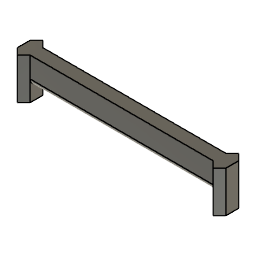
card-dispenser (Autodesk Fusion 360 archive; units mm, degrees)
design "dispenser-gate"
part number: 2026-07-27-01-31-44-288
Autodesk Fusion 360 part; units mm, degrees
(part 1 of 3)
sketch "Sketch1" plane through (0, 0, 0) normal (0, 0, 1) x (1, 0, 0)
  line L0 (0, 5) -> (5, 5)
  line L1 (5, 5) -> (5, 0)
  line L2 (5, 0) -> (0, 0)
  line L3 (0, 0) -> (0, 5)
  line L4 (0, 5) -> (2.5, 7.5)
  line L5 (2.5, 7.5) -> (5, 5)
  line L6 (0, 0) -> (2.5, -2.5)
  line L7 (2.5, -2.5) -> (5, 0)
  line L8 (0, 0) -> (81, 0)
  line L9 (81, 0) -> (81, 5)
  line L10 (81, 5) -> (0, 5)
  line L11 (81, 5) -> (76, 5)
  line L12 (76, 5) -> (76, 0)
  line L13 (76, 5) -> (78.5, 7.5)
  line L14 (78.5, 7.5) -> (81, 5)
  line L15 (81, 0) -> (78.5, -2.5)
  line L16 (76, 0) -> (78.5, -2.5)
  constraint horizontal L0
  constraint vertical L1
  constraint horizontal L2
  constraint vertical L3
  constraint perpendicular L4 L5
  constraint coincident L2.end L3.start
  constraint parallel L5 L6
  constraint perpendicular L6 L7
  constraint perpendicular L3 L8
  constraint perpendicular L2 L9
  constraint perpendicular L3 L10
  constraint coincident L10 L11.end
  constraint coincident L8 L12.end
  constraint perpendicular L8 L12
  constraint perpendicular L13 L14
  constraint perpendicular L14 L15
  constraint perpendicular L15 L16
extrude "Extrude1" add sketch "Sketch1" along normal blind 16
sketch "Sketch2" plane through (0, 0, 0) normal (0, -1, 0) x (1, 0, 0)
  line L0 (5, 0) -> (76, 0)
  line L1 (76, 0) -> (76, 16)
  line L2 (76, 16) -> (5, 16)
  line L3 (5, 16) -> (5, 0)
  line L4 (5, 0) -> (76, 0)
  line L5 (76, 0) -> (76, 5.45)
  line L6 (76, 5.45) -> (5, 5.45)
  line L7 (5, 5.45) -> (5, 0)
  dimension "d3" = 71
  dimension "d4" = 5.45
  constraint horizontal L4
  constraint vertical L5
  constraint horizontal L6
  constraint vertical L7
  constraint coincident L0.start L3.end
  measures "d3" distance of L0.start L0.end
  measures "d4" distance of L0.start L6.end
extrude "Extrude2" cut sketch "Sketch2" against normal blind 5 contours L0 L1 L3 L4 L5 L6 L7
fillet "Fillet1" radius 2.5 2 edges at (40.5, 0, 5.45) (40.5, 5, 5.45)

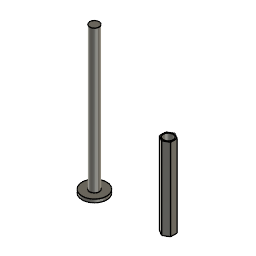
design "card-dispenser-shaft"
part number: 2026-07-26-23-05-58-167
part number: 2026-07-27-03-40-20-627
part number: 2026-07-27-03-40-25-472
Autodesk Fusion 360 part; units mm, degrees
sketch "Sketch1" plane through (0, 0, 0) normal (0, 0, 1) x (1, 0, 0)
  circle A0 centre (0, 0) radius 2.9
  circle A1 centre (0, 0) radius 7.5
  circle A2 centre (45, 0) radius 2.95
  line L0 (45, 4) -> (41.5359, 2)
  line L1 (41.5359, 2) -> (41.5359, -2)
  line L2 (41.5359, -2) -> (45, -4)
  line L3 (45, -4) -> (48.4641, -2)
  line L4 (48.4641, -2) -> (48.4641, 2)
  line L5 (48.4641, 2) -> (45, 4)
  point P0 (45, 0)
  point P1 (45, 0)
  dimension "d1" = 5.8
  dimension "d4" = 15
  dimension "d7" = 5.9
  constraint coincident A0.centre A1.centre
  constraint concentric A0 A1
  constraint coincident P1 P0
  measures "d1" diameter of A0
  measures "d4" diameter of A1
  measures "d7" diameter of A2
extrude "Extrude1" add sketch "Sketch1" along normal blind 87 contours A0 makes body 1
extrude "Extrude2" add sketch "Sketch1" against normal blind 2 contours A0 | A1 bodies 1
extrude "Extrude3" add sketch "Sketch1" along normal blind 50 separate body contours L0 L1 L2 L3 L4 L5 makes body 2
copy_body "Body->Comp1" bodies 2 removing the originals makes body 3 in component "Component"
copy_body "Body->Comp2" bodies 1 removing the originals makes body 4 in component "Component'"
component "Component" placed x (1, 0, 0) y (0, 1, 0) z (0, 0, 1) at (0, 0, 0)
component "Component'" placed x (1, 0, 0) y (0, 1, 0) z (0, 0, 1) at (0, 0, 0)

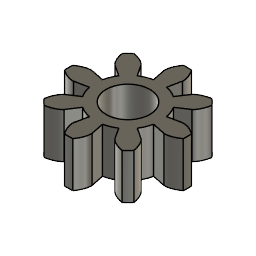
design "dispenser-driven-gear"
part number: 2026-07-25-20-51-35-213
part number: 2026-07-27-03-07-20-434
Autodesk Fusion 360 part; units mm, degrees
sketch "Sketch1" plane through (0, 0, 0) normal (0, 0, 1) x (1, 0, 0) in component "Component"
  spline S0 degree 5 poles (6.0079, -1.2297) (6.008, -1.2297) (6.0082, -1.2298) (6.0085, -1.2298) (6.009, -1.2299) (6.0098, -1.23) (6.0106, -1.2302) (6.0116, -1.2304) (6.0127, -1.2305) (6.0139, -1.2307) (6.0152, -1.2309) (6.0166, -1.2311) (6.0182, -1.2314) (6.0198, -1.2316) (6.0216, -1.2318) (6.0234, -1.2321) (6.0254, -1.2323) (6.0274, -1.2326) (6.0296, -1.2328) (6.0318, -1.2331) (6.0342, -1.2333) (6.0366, -1.2336) (6.0392, -1.2339) (6.0418, -1.2341) (6.0446, -1.2344) (6.0474, -1.2346) (6.0503, -1.2349) (6.0533, -1.2351) (6.0564, -1.2353) (6.0596, -1.2356) (6.0629, -1.2358) (6.0663, -1.236) (6.0698, -1.2362) (6.0733, -1.2364) (6.077, -1.2366) (6.0807, -1.2368) (6.0845, -1.237) (6.0884, -1.2371) (6.0923, -1.2373) (6.0964, -1.2374) (6.1005, -1.2375) (6.1047, -1.2376) (6.109, -1.2377) (6.1134, -1.2378) (6.1179, -1.2379) (6.1224, -1.2379) (6.127, -1.2379) (6.1317, -1.2379) (6.1364, -1.2379) (6.1413, -1.2379) (6.1462, -1.2379) (6.1511, -1.2378) (6.1562, -1.2377) (6.1613, -1.2376) (6.1665, -1.2375) (6.1718, -1.2373) (6.1771, -1.2372) (6.1825, -1.237) (6.188, -1.2367) (6.1935, -1.2365) (6.1991, -1.2362) (6.2048, -1.236) (6.2105, -1.2356) (6.2163, -1.2353) (6.2222, -1.2349) (6.2281, -1.2346) (6.2341, -1.2341) (6.2402, -1.2337) (6.2463, -1.2332) (6.2525, -1.2327) (6.2587, -1.2322) (6.265, -1.2317) (6.2714, -1.2311) (6.2778, -1.2305) (6.2843, -1.2299) (6.2909, -1.2292) (6.2975, -1.2285) (6.3041, -1.2278) (6.3109, -1.227) (6.3176, -1.2262) (6.3245, -1.2254) (6.3314, -1.2246) (6.3383, -1.2237) (6.3453, -1.2228) (6.3524, -1.2219) (6.3595, -1.2209) (6.3666, -1.2199) (6.3739, -1.2188) (6.3811, -1.2178) (6.3885, -1.2167) (6.3958, -1.2155) (6.4033, -1.2144) (6.4107, -1.2131) (6.4183, -1.2119) (6.4258, -1.2106) (6.4335, -1.2093) (6.4411, -1.208) (6.4489, -1.2066) (6.4566, -1.2052) (6.4645, -1.2037) (6.4723, -1.2022) (6.4802, -1.2007) (6.4882, -1.1991) (6.4962, -1.1975) (6.5043, -1.1959) (6.5124, -1.1942) (6.5205, -1.1925) (6.5287, -1.1908) (6.5369, -1.189) (6.5452, -1.1872) (6.5535, -1.1853) (6.5619, -1.1834) (6.5703, -1.1814) (6.5787, -1.1795) (6.5872, -1.1774) (6.5957, -1.1754) (6.6043, -1.1733) (6.6129, -1.1712) (6.6216, -1.169) (6.6302, -1.1668) (6.639, -1.1645) (6.6477, -1.1622) (6.6565, -1.1599) (6.6654, -1.1575) (6.6743, -1.1551) (6.6832, -1.1526) (6.6921, -1.1501) (6.7011, -1.1476) (6.7102, -1.145) (6.7192, -1.1424) (6.7283, -1.1397) (6.7375, -1.137) (6.7466, -1.1342) (6.7558, -1.1314) (6.7651, -1.1286) (6.7744, -1.1257) (6.7837, -1.1228) (6.793, -1.1199) (6.8024, -1.1168) (6.8118, -1.1138) (6.8212, -1.1107) (6.8307, -1.1076) (6.8402, -1.1044) (6.8497, -1.1012) (6.8593, -1.0979) (6.8689, -1.0946) (6.8785, -1.0913) (6.8881, -1.0879) (6.8978, -1.0844) (6.9075, -1.0809) (6.9173, -1.0774) (6.927, -1.0738) (6.9368, -1.0702) (6.9467, -1.0666) (6.9565, -1.0628) (6.9664, -1.0591) (6.9763, -1.0553) (6.9862, -1.0515) (6.9962, -1.0476) (7.0062, -1.0436) (7.0162, -1.0397) (7.0262, -1.0356) (7.0363, -1.0316) (7.0464, -1.0275) (7.0565, -1.0233) (7.0666, -1.0191) (7.0768, -1.0149) (7.087, -1.0106) (7.0972, -1.0062) (7.1074, -1.0018) (7.1176, -0.9974) (7.1279, -0.9929) (7.1382, -0.9884) (7.1485, -0.9838) (7.1589, -0.9792) (7.1692, -0.9745) (7.1796, -0.9698) (7.19, -0.9651) (7.2004, -0.9603) (7.2109, -0.9554) (7.2213, -0.9505) (7.2318, -0.9456) (7.2423, -0.9406) (7.2528, -0.9356) (7.2634, -0.9305) (7.2739, -0.9253) (7.2845, -0.9202) (7.2951, -0.9149) (7.3057, -0.9097) (7.3163, -0.9044) (7.327, -0.899) (7.3376, -0.8936) (7.3483, -0.8881) (7.359, -0.8826) (7.3697, -0.8771) (7.3804, -0.8714) (7.3912, -0.8658) (7.4019, -0.8601) (7.4127, -0.8544) (7.4235, -0.8486) (7.4343, -0.8427) (7.4451, -0.8368) (7.4559, -0.8309) (7.4667, -0.8249) (7.4776, -0.8189) (7.4885, -0.8128) (7.4993, -0.8067) (7.5102, -0.8005) (7.5211, -0.7943) (7.532, -0.788) (7.543, -0.7817) (7.5539, -0.7753) (7.5648, -0.7689) (7.5758, -0.7624) (7.5868, -0.7559) (7.5978, -0.7494) (7.6087, -0.7428) (7.6197, -0.7361) (7.6308, -0.7294) (7.6418, -0.7226) (7.6528, -0.7158) (7.6638, -0.709) (7.6749, -0.7021) (7.6859, -0.6951) (7.697, -0.6882) (7.7081, -0.6811) (7.7192, -0.674) (7.7302, -0.6669) (7.7413, -0.6597) (7.7524, -0.6525) (7.7635, -0.6452) (7.7746, -0.6378) (7.7858, -0.6305) (7.7969, -0.623) (7.808, -0.6156) (7.8192, -0.608) (7.8303, -0.6005) (7.8415, -0.5928) (7.8526, -0.5852) (7.8638, -0.5774) (7.8749, -0.5697) (7.8839, -0.5634) (7.8906, -0.5587) (7.895, -0.5556) (7.8973, -0.554) knots 0 0 0 0 0 0 0.00416667 0.00833333 0.0125 0.01666667 0.02083333 0.025 0.02916667 0.03333333 0.0375 0.04166667 0.04583333 0.05 0.05416667 0.05833333 0.0625 0.06666667 0.07083333 0.075 0.07916667 0.08333333 0.0875 0.09166667 0.09583333 0.1 0.10416667 0.10833333 0.1125 0.11666667 0.12083333 0.125 0.12916667 0.13333333 0.1375 0.14166667 0.14583333 0.15 0.15416667 0.15833333 0.1625 0.16666667 0.17083333 0.175 0.17916667 0.18333333 0.1875 0.19166667 0.19583333 0.2 0.20416667 0.20833333 0.2125 0.21666667 0.22083333 0.225 0.22916667 0.23333333 0.2375 0.24166667 0.24583333 0.25 0.25416667 0.25833333 0.2625 0.26666667 0.27083333 0.275 0.27916667 0.28333333 0.2875 0.29166667 0.29583333 0.3 0.30416667 0.30833333 0.3125 0.31666667 0.32083333 0.325 0.32916667 0.33333333 0.3375 0.34166667 0.34583333 0.35 0.35416667 0.35833333 0.3625 0.36666667 0.37083333 0.375 0.37916667 0.38333333 0.3875 0.39166667 0.39583333 0.4 0.40416667 0.40833333 0.4125 0.41666667 0.42083333 0.425 0.42916667 0.43333333 0.4375 0.44166667 0.44583333 0.45 0.45416667 0.45833333 0.4625 0.46666667 0.47083333 0.475 0.47916667 0.48333333 0.4875 0.49166667 0.49583333 0.5 0.50416667 0.50833333 0.5125 0.51666667 0.52083333 0.525 0.52916667 0.53333333 0.5375 0.54166667 0.54583333 0.55 0.55416667 0.55833333 0.5625 0.56666667 0.57083333 0.575 0.57916667 0.58333333 0.5875 0.59166667 0.59583333 0.6 0.60416667 0.60833333 0.6125 0.61666667 0.62083333 0.625 0.62916667 0.63333333 0.6375 0.64166667 0.64583333 0.65 0.65416667 0.65833333 0.6625 0.66666667 0.67083333 0.675 0.67916667 0.68333333 0.6875 0.69166667 0.69583333 0.7 0.70416667 0.70833333 0.7125 0.71666667 0.72083333 0.725 0.72916667 0.73333333 0.7375 0.74166667 0.74583333 0.75 0.75416667 0.75833333 0.7625 0.76666667 0.77083333 0.775 0.77916667 0.78333333 0.7875 0.79166667 0.79583333 0.8 0.80416667 0.80833333 0.8125 0.81666667 0.82083333 0.825 0.82916667 0.83333333 0.8375 0.84166667 0.84583333 0.85 0.85416667 0.85833333 0.8625 0.86666667 0.87083333 0.875 0.87916667 0.88333333 0.8875 0.89166667 0.89583333 0.9 0.90416667 0.90833333 0.9125 0.91666667 0.92083333 0.925 0.92916667 0.93333333 0.9375 0.94166667 0.94583333 0.95 0.95416667 0.95833333 0.9625 0.96666667 0.97083333 0.975 0.97916667 0.98333333 0.9875 0.99166667 0.99583333 1 1 1 1 1 1
  spline S1 degree 5 poles (6.0079, 1.2297) (6.008, 1.2297) (6.0082, 1.2298) (6.0085, 1.2298) (6.009, 1.2299) (6.0098, 1.23) (6.0106, 1.2302) (6.0116, 1.2304) (6.0127, 1.2305) (6.0139, 1.2307) (6.0152, 1.2309) (6.0166, 1.2311) (6.0182, 1.2314) (6.0198, 1.2316) (6.0216, 1.2318) (6.0234, 1.2321) (6.0254, 1.2323) (6.0274, 1.2326) (6.0296, 1.2328) (6.0318, 1.2331) (6.0342, 1.2333) (6.0366, 1.2336) (6.0392, 1.2339) (6.0418, 1.2341) (6.0446, 1.2344) (6.0474, 1.2346) (6.0503, 1.2349) (6.0533, 1.2351) (6.0564, 1.2353) (6.0596, 1.2356) (6.0629, 1.2358) (6.0663, 1.236) (6.0698, 1.2362) (6.0733, 1.2364) (6.077, 1.2366) (6.0807, 1.2368) (6.0845, 1.237) (6.0884, 1.2371) (6.0923, 1.2373) (6.0964, 1.2374) (6.1005, 1.2375) (6.1047, 1.2376) (6.109, 1.2377) (6.1134, 1.2378) (6.1179, 1.2379) (6.1224, 1.2379) (6.127, 1.2379) (6.1317, 1.2379) (6.1364, 1.2379) (6.1413, 1.2379) (6.1462, 1.2379) (6.1511, 1.2378) (6.1562, 1.2377) (6.1613, 1.2376) (6.1665, 1.2375) (6.1718, 1.2373) (6.1771, 1.2372) (6.1825, 1.237) (6.188, 1.2367) (6.1935, 1.2365) (6.1991, 1.2362) (6.2048, 1.236) (6.2105, 1.2356) (6.2163, 1.2353) (6.2222, 1.2349) (6.2281, 1.2346) (6.2341, 1.2341) (6.2402, 1.2337) (6.2463, 1.2332) (6.2525, 1.2327) (6.2587, 1.2322) (6.265, 1.2317) (6.2714, 1.2311) (6.2778, 1.2305) (6.2843, 1.2299) (6.2909, 1.2292) (6.2975, 1.2285) (6.3041, 1.2278) (6.3109, 1.227) (6.3176, 1.2262) (6.3245, 1.2254) (6.3314, 1.2246) (6.3383, 1.2237) (6.3453, 1.2228) (6.3524, 1.2219) (6.3595, 1.2209) (6.3666, 1.2199) (6.3739, 1.2188) (6.3811, 1.2178) (6.3885, 1.2167) (6.3958, 1.2155) (6.4033, 1.2144) (6.4107, 1.2131) (6.4183, 1.2119) (6.4258, 1.2106) (6.4335, 1.2093) (6.4411, 1.208) (6.4489, 1.2066) (6.4566, 1.2052) (6.4645, 1.2037) (6.4723, 1.2022) (6.4802, 1.2007) (6.4882, 1.1991) (6.4962, 1.1975) (6.5043, 1.1959) (6.5124, 1.1942) (6.5205, 1.1925) (6.5287, 1.1908) (6.5369, 1.189) (6.5452, 1.1872) (6.5535, 1.1853) (6.5619, 1.1834) (6.5703, 1.1814) (6.5787, 1.1795) (6.5872, 1.1774) (6.5957, 1.1754) (6.6043, 1.1733) (6.6129, 1.1712) (6.6216, 1.169) (6.6302, 1.1668) (6.639, 1.1645) (6.6477, 1.1622) (6.6565, 1.1599) (6.6654, 1.1575) (6.6743, 1.1551) (6.6832, 1.1526) (6.6921, 1.1501) (6.7011, 1.1476) (6.7102, 1.145) (6.7192, 1.1424) (6.7283, 1.1397) (6.7375, 1.137) (6.7466, 1.1342) (6.7558, 1.1314) (6.7651, 1.1286) (6.7744, 1.1257) (6.7837, 1.1228) (6.793, 1.1199) (6.8024, 1.1168) (6.8118, 1.1138) (6.8212, 1.1107) (6.8307, 1.1076) (6.8402, 1.1044) (6.8497, 1.1012) (6.8593, 1.0979) (6.8689, 1.0946) (6.8785, 1.0913) (6.8881, 1.0879) (6.8978, 1.0844) (6.9075, 1.0809) (6.9173, 1.0774) (6.927, 1.0738) (6.9368, 1.0702) (6.9467, 1.0666) (6.9565, 1.0628) (6.9664, 1.0591) (6.9763, 1.0553) (6.9862, 1.0515) (6.9962, 1.0476) (7.0062, 1.0436) (7.0162, 1.0397) (7.0262, 1.0356) (7.0363, 1.0316) (7.0464, 1.0275) (7.0565, 1.0233) (7.0666, 1.0191) (7.0768, 1.0149) (7.087, 1.0106) (7.0972, 1.0062) (7.1074, 1.0018) (7.1176, 0.9974) (7.1279, 0.9929) (7.1382, 0.9884) (7.1485, 0.9838) (7.1589, 0.9792) (7.1692, 0.9745) (7.1796, 0.9698) (7.19, 0.9651) (7.2004, 0.9603) (7.2109, 0.9554) (7.2213, 0.9505) (7.2318, 0.9456) (7.2423, 0.9406) (7.2528, 0.9356) (7.2634, 0.9305) (7.2739, 0.9253) (7.2845, 0.9202) (7.2951, 0.9149) (7.3057, 0.9097) (7.3163, 0.9044) (7.327, 0.899) (7.3376, 0.8936) (7.3483, 0.8881) (7.359, 0.8826) (7.3697, 0.8771) (7.3804, 0.8714) (7.3912, 0.8658) (7.4019, 0.8601) (7.4127, 0.8544) (7.4235, 0.8486) (7.4343, 0.8427) (7.4451, 0.8368) (7.4559, 0.8309) (7.4667, 0.8249) (7.4776, 0.8189) (7.4885, 0.8128) (7.4993, 0.8067) (7.5102, 0.8005) (7.5211, 0.7943) (7.532, 0.788) (7.543, 0.7817) (7.5539, 0.7753) (7.5648, 0.7689) (7.5758, 0.7624) (7.5868, 0.7559) (7.5978, 0.7494) (7.6087, 0.7428) (7.6197, 0.7361) (7.6308, 0.7294) (7.6418, 0.7226) (7.6528, 0.7158) (7.6638, 0.709) (7.6749, 0.7021) (7.6859, 0.6951) (7.697, 0.6882) (7.7081, 0.6811) (7.7192, 0.674) (7.7302, 0.6669) (7.7413, 0.6597) (7.7524, 0.6525) (7.7635, 0.6452) (7.7746, 0.6378) (7.7858, 0.6305) (7.7969, 0.623) (7.808, 0.6156) (7.8192, 0.608) (7.8303, 0.6005) (7.8415, 0.5928) (7.8526, 0.5852) (7.8638, 0.5774) (7.8749, 0.5697) (7.8839, 0.5634) (7.8906, 0.5587) (7.895, 0.5556) (7.8973, 0.554) knots 0 0 0 0 0 0 0.00416667 0.00833333 0.0125 0.01666667 0.02083333 0.025 0.02916667 0.03333333 0.0375 0.04166667 0.04583333 0.05 0.05416667 0.05833333 0.0625 0.06666667 0.07083333 0.075 0.07916667 0.08333333 0.0875 0.09166667 0.09583333 0.1 0.10416667 0.10833333 0.1125 0.11666667 0.12083333 0.125 0.12916667 0.13333333 0.1375 0.14166667 0.14583333 0.15 0.15416667 0.15833333 0.1625 0.16666667 0.17083333 0.175 0.17916667 0.18333333 0.1875 0.19166667 0.19583333 0.2 0.20416667 0.20833333 0.2125 0.21666667 0.22083333 0.225 0.22916667 0.23333333 0.2375 0.24166667 0.24583333 0.25 0.25416667 0.25833333 0.2625 0.26666667 0.27083333 0.275 0.27916667 0.28333333 0.2875 0.29166667 0.29583333 0.3 0.30416667 0.30833333 0.3125 0.31666667 0.32083333 0.325 0.32916667 0.33333333 0.3375 0.34166667 0.34583333 0.35 0.35416667 0.35833333 0.3625 0.36666667 0.37083333 0.375 0.37916667 0.38333333 0.3875 0.39166667 0.39583333 0.4 0.40416667 0.40833333 0.4125 0.41666667 0.42083333 0.425 0.42916667 0.43333333 0.4375 0.44166667 0.44583333 0.45 0.45416667 0.45833333 0.4625 0.46666667 0.47083333 0.475 0.47916667 0.48333333 0.4875 0.49166667 0.49583333 0.5 0.50416667 0.50833333 0.5125 0.51666667 0.52083333 0.525 0.52916667 0.53333333 0.5375 0.54166667 0.54583333 0.55 0.55416667 0.55833333 0.5625 0.56666667 0.57083333 0.575 0.57916667 0.58333333 0.5875 0.59166667 0.59583333 0.6 0.60416667 0.60833333 0.6125 0.61666667 0.62083333 0.625 0.62916667 0.63333333 0.6375 0.64166667 0.64583333 0.65 0.65416667 0.65833333 0.6625 0.66666667 0.67083333 0.675 0.67916667 0.68333333 0.6875 0.69166667 0.69583333 0.7 0.70416667 0.70833333 0.7125 0.71666667 0.72083333 0.725 0.72916667 0.73333333 0.7375 0.74166667 0.74583333 0.75 0.75416667 0.75833333 0.7625 0.76666667 0.77083333 0.775 0.77916667 0.78333333 0.7875 0.79166667 0.79583333 0.8 0.80416667 0.80833333 0.8125 0.81666667 0.82083333 0.825 0.82916667 0.83333333 0.8375 0.84166667 0.84583333 0.85 0.85416667 0.85833333 0.8625 0.86666667 0.87083333 0.875 0.87916667 0.88333333 0.8875 0.89166667 0.89583333 0.9 0.90416667 0.90833333 0.9125 0.91666667 0.92083333 0.925 0.92916667 0.93333333 0.9375 0.94166667 0.94583333 0.95 0.95416667 0.95833333 0.9625 0.96666667 0.97083333 0.975 0.97916667 0.98333333 0.9875 0.99166667 0.99583333 1 1 1 1 1 1
  spline S2 degree 5 poles (6.0071, -1.2295) (6.0071, -1.2295) (6.0072, -1.2296) (6.0073, -1.2296) (6.0074, -1.2296) (6.0076, -1.2296) (6.0077, -1.2297) (6.0078, -1.2297) (6.0079, -1.2297) (6.0079, -1.2297) knots 0 0 0 0 0 0 0.2 0.4 0.6 0.8 1 1 1 1 1 1
  spline S3 degree 5 poles (6.0071, 1.2295) (6.0071, 1.2295) (6.0072, 1.2296) (6.0073, 1.2296) (6.0074, 1.2296) (6.0076, 1.2296) (6.0077, 1.2297) (6.0078, 1.2297) (6.0079, 1.2297) (6.0079, 1.2297) knots 0 0 0 0 0 0 0.2 0.4 0.6 0.8 1 1 1 1 1 1
  line L0 (0, 0) -> (6.0071, -1.2295)
  line L1 (0, 0) -> (6.0071, 1.2295)
  arc A0 (7.8973, -0.554) -> (7.8973, 0.554) centre (0, 0) ccw
  point P0 (6.0104, -1.2302)
  point P1 (6.0146, -1.2308)
  point P2 (6.0205, -1.2317)
  point P3 (6.0281, -1.2326)
  point P4 (6.0374, -1.2337)
  point P5 (6.0485, -1.2347)
  point P6 (6.0612, -1.2357)
  point P7 (6.0756, -1.2366)
  point P8 (6.0918, -1.2373)
  point P9 (6.1097, -1.2377)
  point P10 (6.1293, -1.2379)
  point P11 (6.1506, -1.2378)
  point P12 (6.1736, -1.2373)
  point P13 (6.1982, -1.2363)
  point P14 (6.2246, -1.2348)
  point P15 (6.2526, -1.2327)
  point P16 (6.2823, -1.2301)
  point P17 (6.3137, -1.2267)
  point P18 (6.3466, -1.2226)
  point P19 (6.3812, -1.2178)
  point P20 (6.4174, -1.212)
  point P21 (6.4551, -1.2054)
  point P22 (6.4944, -1.1979)
  point P23 (6.5353, -1.1893)
  point P24 (6.5776, -1.1797)
  point P25 (6.6215, -1.169)
  point P26 (6.6668, -1.1571)
  point P27 (6.7135, -1.144)
  point P28 (6.7617, -1.1296)
  point P29 (6.8112, -1.114)
  point P30 (6.8621, -1.0969)
  point P31 (6.9143, -1.0785)
  point P32 (6.9678, -1.0586)
  point P33 (7.0225, -1.0371)
  point P34 (7.0784, -1.0142)
  point P35 (7.1355, -0.9896)
  point P36 (7.1938, -0.9633)
  point P37 (7.2531, -0.9354)
  point P38 (7.3135, -0.9058)
  point P39 (7.3749, -0.8743)
  point P40 (7.4373, -0.8411)
  point P41 (7.5006, -0.806)
  point P42 (7.5648, -0.7689)
  point P43 (7.6298, -0.73)
  point P44 (7.6956, -0.689)
  point P45 (7.7621, -0.6461)
  point P46 (7.8294, -0.6011)
  point P47 (6.0104, 1.2302)
  point P48 (6.0146, 1.2308)
  point P49 (6.0205, 1.2317)
  point P50 (6.0281, 1.2326)
  point P51 (6.0374, 1.2337)
  point P52 (6.0485, 1.2347)
  point P53 (6.0612, 1.2357)
  point P54 (6.0756, 1.2366)
  point P55 (6.0918, 1.2373)
  point P56 (6.1097, 1.2377)
  point P57 (6.1293, 1.2379)
  point P58 (6.1506, 1.2378)
  point P59 (6.1736, 1.2373)
  point P60 (6.1982, 1.2363)
  point P61 (6.2246, 1.2348)
  point P62 (6.2526, 1.2327)
  point P63 (6.2823, 1.2301)
  point P64 (6.3137, 1.2267)
  point P65 (6.3466, 1.2226)
  point P66 (6.3812, 1.2178)
  point P67 (6.4174, 1.212)
  point P68 (6.4551, 1.2054)
  point P69 (6.4944, 1.1979)
  point P70 (6.5353, 1.1893)
  point P71 (6.5776, 1.1797)
  point P72 (6.6215, 1.169)
  point P73 (6.6668, 1.1571)
  point P74 (6.7135, 1.144)
  point P75 (6.7617, 1.1296)
  point P76 (6.8112, 1.114)
  point P77 (6.8621, 1.0969)
  point P78 (6.9143, 1.0785)
  point P79 (6.9678, 1.0586)
  point P80 (7.0225, 1.0371)
  point P81 (7.0784, 1.0142)
  point P82 (7.1355, 0.9896)
  point P83 (7.1938, 0.9633)
  point P84 (7.2531, 0.9354)
  point P85 (7.3135, 0.9058)
  point P86 (7.3749, 0.8743)
  point P87 (7.4373, 0.8411)
  point P88 (7.5006, 0.806)
  point P89 (7.5648, 0.7689)
  point P90 (7.6298, 0.73)
  point P91 (7.6956, 0.689)
  point P92 (7.7621, 0.6461)
  point P93 (7.8294, 0.6011)
sketch "Sketch2" plane through (0, 0, 0) normal (0, 0, 1) x (1, 0, 0) in component "Component"
  circle A0 centre (0, 0) radius 4.3542
extrude "Extrude1" add sketch "Sketch2" along normal blind 6 makes body 1 in component "Component"
extrude "Extrude2" add sketch "Sketch1" along normal blind 6 separate body makes body 2 in component "Component"
pattern_circular "C-Pattern1" count 8 over 360 about axis through (0, 0, 1.75) along (0, 0, 1) of "Extrude2" makes body 3 at (1.7059, 1.1262, 2) makes body 4 at (0.4099, 2.0026, 2) makes body 5 at (-1.1262, 1.7059, 2) makes body 6 at (-2.0026, 0.4099, 2) makes body 7 at (-1.1262, -1.7059, 2) makes body 8 at (-0.4099, -2.0026, 2) makes body 9 at (1.1262, -1.7059, 2) in component "Component"
combine "Combine1" operation add target body 1 tool bodies 2 3 4 5 6 7 8 9 in component "Component"
sketch "Sketch3" plane through (0, 0, 0) normal (0, 0, 1) x (1, 0, 0) in component "Component"
  line L0 (0, 0) -> (59.7744, 0) construction
  line L1 (59.7744, 0) -> (59.7744, 3) construction
  line L2 (59.7744, 3) -> (0, 3) construction
  line L3 (0, 3) -> (0, 0) construction
  constraint perpendicular L0 L1
  constraint parallel L0 L2
  constraint parallel L1 L3
sketch "Sketch3 (2)" plane through (0, 0, 6) normal (0, 0, 1) x (-1, 0, 0)
  arc A0 (-3.6337, 2.3989) -> (-4.2657, 0.8731) centre (0, 0) ccw
  line L0 (-4.2657, 0.8731) -> (-6.0071, 1.2295)
  line L1 (-6.0071, 1.2295) -> (-6.0079, 1.2297)
  spline S0 degree 5 poles (-6.0079, 1.2297) (-6.008, 1.2297) (-6.0082, 1.2298) (-6.0085, 1.2298) (-6.009, 1.2299) (-6.0098, 1.23) (-6.0106, 1.2302) (-6.0116, 1.2304) (-6.0127, 1.2305) (-6.0139, 1.2307) (-6.0152, 1.2309) (-6.0166, 1.2311) (-6.0182, 1.2314) (-6.0198, 1.2316) (-6.0216, 1.2318) (-6.0234, 1.2321) (-6.0254, 1.2323) (-6.0274, 1.2326) (-6.0296, 1.2328) (-6.0318, 1.2331) (-6.0342, 1.2333) (-6.0366, 1.2336) (-6.0392, 1.2339) (-6.0418, 1.2341) (-6.0446, 1.2344) (-6.0474, 1.2346) (-6.0503, 1.2349) (-6.0533, 1.2351) (-6.0564, 1.2353) (-6.0596, 1.2356) (-6.0629, 1.2358) (-6.0663, 1.236) (-6.0698, 1.2362) (-6.0733, 1.2364) (-6.077, 1.2366) (-6.0807, 1.2368) (-6.0845, 1.237) (-6.0884, 1.2371) (-6.0923, 1.2373) (-6.0964, 1.2374) (-6.1005, 1.2375) (-6.1047, 1.2376) (-6.109, 1.2377) (-6.1134, 1.2378) (-6.1179, 1.2379) (-6.1224, 1.2379) (-6.127, 1.2379) (-6.1317, 1.2379) (-6.1364, 1.2379) (-6.1413, 1.2379) (-6.1462, 1.2379) (-6.1511, 1.2378) (-6.1562, 1.2377) (-6.1613, 1.2376) (-6.1665, 1.2375) (-6.1718, 1.2373) (-6.1771, 1.2372) (-6.1825, 1.237) (-6.188, 1.2367) (-6.1935, 1.2365) (-6.1991, 1.2362) (-6.2048, 1.236) (-6.2105, 1.2356) (-6.2163, 1.2353) (-6.2222, 1.2349) (-6.2281, 1.2346) (-6.2341, 1.2341) (-6.2402, 1.2337) (-6.2463, 1.2332) (-6.2525, 1.2327) (-6.2587, 1.2322) (-6.265, 1.2317) (-6.2714, 1.2311) (-6.2778, 1.2305) (-6.2843, 1.2299) (-6.2909, 1.2292) (-6.2975, 1.2285) (-6.3041, 1.2278) (-6.3109, 1.227) (-6.3176, 1.2262) (-6.3245, 1.2254) (-6.3314, 1.2246) (-6.3383, 1.2237) (-6.3453, 1.2228) (-6.3524, 1.2219) (-6.3595, 1.2209) (-6.3666, 1.2199) (-6.3739, 1.2188) (-6.3811, 1.2178) (-6.3885, 1.2167) (-6.3958, 1.2155) (-6.4033, 1.2144) (-6.4107, 1.2131) (-6.4183, 1.2119) (-6.4258, 1.2106) (-6.4335, 1.2093) (-6.4411, 1.208) (-6.4489, 1.2066) (-6.4566, 1.2052) (-6.4645, 1.2037) (-6.4723, 1.2022) (-6.4802, 1.2007) (-6.4882, 1.1991) (-6.4962, 1.1975) (-6.5043, 1.1959) (-6.5124, 1.1942) (-6.5205, 1.1925) (-6.5287, 1.1908) (-6.5369, 1.189) (-6.5452, 1.1872) (-6.5535, 1.1853) (-6.5619, 1.1834) (-6.5703, 1.1814) (-6.5787, 1.1795) (-6.5872, 1.1774) (-6.5957, 1.1754) (-6.6043, 1.1733) (-6.6129, 1.1712) (-6.6216, 1.169) (-6.6302, 1.1668) (-6.639, 1.1645) (-6.6477, 1.1622) (-6.6565, 1.1599) (-6.6654, 1.1575) (-6.6743, 1.1551) (-6.6832, 1.1526) (-6.6921, 1.1501) (-6.7011, 1.1476) (-6.7102, 1.145) (-6.7192, 1.1424) (-6.7283, 1.1397) (-6.7375, 1.137) (-6.7466, 1.1342) (-6.7558, 1.1314) (-6.7651, 1.1286) (-6.7744, 1.1257) (-6.7837, 1.1228) (-6.793, 1.1199) (-6.8024, 1.1168) (-6.8118, 1.1138) (-6.8212, 1.1107) (-6.8307, 1.1076) (-6.8402, 1.1044) (-6.8497, 1.1012) (-6.8593, 1.0979) (-6.8689, 1.0946) (-6.8785, 1.0913) (-6.8881, 1.0879) (-6.8978, 1.0844) (-6.9075, 1.0809) (-6.9173, 1.0774) (-6.927, 1.0738) (-6.9368, 1.0702) (-6.9467, 1.0666) (-6.9565, 1.0628) (-6.9664, 1.0591) (-6.9763, 1.0553) (-6.9862, 1.0515) (-6.9962, 1.0476) (-7.0062, 1.0436) (-7.0162, 1.0397) (-7.0262, 1.0356) (-7.0363, 1.0316) (-7.0464, 1.0275) (-7.0565, 1.0233) (-7.0666, 1.0191) (-7.0768, 1.0149) (-7.087, 1.0106) (-7.0972, 1.0062) (-7.1074, 1.0018) (-7.1176, 0.9974) (-7.1279, 0.9929) (-7.1382, 0.9884) (-7.1485, 0.9838) (-7.1589, 0.9792) (-7.1692, 0.9745) (-7.1796, 0.9698) (-7.19, 0.9651) (-7.2004, 0.9603) (-7.2109, 0.9554) (-7.2213, 0.9505) (-7.2318, 0.9456) (-7.2423, 0.9406) (-7.2528, 0.9356) (-7.2634, 0.9305) (-7.2739, 0.9253) (-7.2845, 0.9202) (-7.2951, 0.9149) (-7.3057, 0.9097) (-7.3163, 0.9044) (-7.327, 0.899) (-7.3376, 0.8936) (-7.3483, 0.8881) (-7.359, 0.8826) (-7.3697, 0.8771) (-7.3804, 0.8714) (-7.3912, 0.8658) (-7.4019, 0.8601) (-7.4127, 0.8544) (-7.4235, 0.8486) (-7.4343, 0.8427) (-7.4451, 0.8368) (-7.4559, 0.8309) (-7.4667, 0.8249) (-7.4776, 0.8189) (-7.4885, 0.8128) (-7.4993, 0.8067) (-7.5102, 0.8005) (-7.5211, 0.7943) (-7.532, 0.788) (-7.543, 0.7817) (-7.5539, 0.7753) (-7.5648, 0.7689) (-7.5758, 0.7624) (-7.5868, 0.7559) (-7.5978, 0.7494) (-7.6087, 0.7428) (-7.6197, 0.7361) (-7.6308, 0.7294) (-7.6418, 0.7226) (-7.6528, 0.7158) (-7.6638, 0.709) (-7.6749, 0.7021) (-7.6859, 0.6951) (-7.697, 0.6882) (-7.7081, 0.6811) (-7.7192, 0.674) (-7.7302, 0.6669) (-7.7413, 0.6597) (-7.7524, 0.6525) (-7.7635, 0.6452) (-7.7746, 0.6378) (-7.7858, 0.6305) (-7.7969, 0.623) (-7.808, 0.6156) (-7.8192, 0.608) (-7.8303, 0.6005) (-7.8415, 0.5928) (-7.8526, 0.5852) (-7.8638, 0.5774) (-7.8749, 0.5697) (-7.8839, 0.5634) (-7.8906, 0.5587) (-7.895, 0.5556) (-7.8973, 0.554) knots 0 0 0 0 0 0 0.00416667 0.00833333 0.0125 0.01666667 0.02083333 0.025 0.02916667 0.03333333 0.0375 0.04166667 0.04583333 0.05 0.05416667 0.05833333 0.0625 0.06666667 0.07083333 0.075 0.07916667 0.08333333 0.0875 0.09166667 0.09583333 0.1 0.10416667 0.10833333 0.1125 0.11666667 0.12083333 0.125 0.12916667 0.13333333 0.1375 0.14166667 0.14583333 0.15 0.15416667 0.15833333 0.1625 0.16666667 0.17083333 0.175 0.17916667 0.18333333 0.1875 0.19166667 0.19583333 0.2 0.20416667 0.20833333 0.2125 0.21666667 0.22083333 0.225 0.22916667 0.23333333 0.2375 0.24166667 0.24583333 0.25 0.25416667 0.25833333 0.2625 0.26666667 0.27083333 0.275 0.27916667 0.28333333 0.2875 0.29166667 0.29583333 0.3 0.30416667 0.30833333 0.3125 0.31666667 0.32083333 0.325 0.32916667 0.33333333 0.3375 0.34166667 0.34583333 0.35 0.35416667 0.35833333 0.3625 0.36666667 0.37083333 0.375 0.37916667 0.38333333 0.3875 0.39166667 0.39583333 0.4 0.40416667 0.40833333 0.4125 0.41666667 0.42083333 0.425 0.42916667 0.43333333 0.4375 0.44166667 0.44583333 0.45 0.45416667 0.45833333 0.4625 0.46666667 0.47083333 0.475 0.47916667 0.48333333 0.4875 0.49166667 0.49583333 0.5 0.50416667 0.50833333 0.5125 0.51666667 0.52083333 0.525 0.52916667 0.53333333 0.5375 0.54166667 0.54583333 0.55 0.55416667 0.55833333 0.5625 0.56666667 0.57083333 0.575 0.57916667 0.58333333 0.5875 0.59166667 0.59583333 0.6 0.60416667 0.60833333 0.6125 0.61666667 0.62083333 0.625 0.62916667 0.63333333 0.6375 0.64166667 0.64583333 0.65 0.65416667 0.65833333 0.6625 0.66666667 0.67083333 0.675 0.67916667 0.68333333 0.6875 0.69166667 0.69583333 0.7 0.70416667 0.70833333 0.7125 0.71666667 0.72083333 0.725 0.72916667 0.73333333 0.7375 0.74166667 0.74583333 0.75 0.75416667 0.75833333 0.7625 0.76666667 0.77083333 0.775 0.77916667 0.78333333 0.7875 0.79166667 0.79583333 0.8 0.80416667 0.80833333 0.8125 0.81666667 0.82083333 0.825 0.82916667 0.83333333 0.8375 0.84166667 0.84583333 0.85 0.85416667 0.85833333 0.8625 0.86666667 0.87083333 0.875 0.87916667 0.88333333 0.8875 0.89166667 0.89583333 0.9 0.90416667 0.90833333 0.9125 0.91666667 0.92083333 0.925 0.92916667 0.93333333 0.9375 0.94166667 0.94583333 0.95 0.95416667 0.95833333 0.9625 0.96666667 0.97083333 0.975 0.97916667 0.98333333 0.9875 0.99166667 0.99583333 1 1 1 1 1 1
  arc A1 (-7.8973, 0.554) -> (-7.8973, -0.554) centre (0, 0) ccw
  spline S1 degree 5 poles (-7.8973, -0.554) (-7.895, -0.5556) (-7.8906, -0.5587) (-7.8839, -0.5634) (-7.8749, -0.5697) (-7.8638, -0.5774) (-7.8526, -0.5852) (-7.8415, -0.5928) (-7.8303, -0.6005) (-7.8192, -0.608) (-7.808, -0.6156) (-7.7969, -0.623) (-7.7858, -0.6305) (-7.7746, -0.6378) (-7.7635, -0.6452) (-7.7524, -0.6525) (-7.7413, -0.6597) (-7.7302, -0.6669) (-7.7192, -0.674) (-7.7081, -0.6811) (-7.697, -0.6882) (-7.6859, -0.6951) (-7.6749, -0.7021) (-7.6638, -0.709) (-7.6528, -0.7158) (-7.6418, -0.7226) (-7.6308, -0.7294) (-7.6197, -0.7361) (-7.6087, -0.7428) (-7.5978, -0.7494) (-7.5868, -0.7559) (-7.5758, -0.7624) (-7.5648, -0.7689) (-7.5539, -0.7753) (-7.543, -0.7817) (-7.532, -0.788) (-7.5211, -0.7943) (-7.5102, -0.8005) (-7.4993, -0.8067) (-7.4885, -0.8128) (-7.4776, -0.8189) (-7.4667, -0.8249) (-7.4559, -0.8309) (-7.4451, -0.8368) (-7.4343, -0.8427) (-7.4235, -0.8486) (-7.4127, -0.8544) (-7.4019, -0.8601) (-7.3912, -0.8658) (-7.3804, -0.8714) (-7.3697, -0.8771) (-7.359, -0.8826) (-7.3483, -0.8881) (-7.3376, -0.8936) (-7.327, -0.899) (-7.3163, -0.9044) (-7.3057, -0.9097) (-7.2951, -0.9149) (-7.2845, -0.9202) (-7.2739, -0.9253) (-7.2634, -0.9305) (-7.2528, -0.9356) (-7.2423, -0.9406) (-7.2318, -0.9456) (-7.2213, -0.9505) (-7.2109, -0.9554) (-7.2004, -0.9603) (-7.19, -0.9651) (-7.1796, -0.9698) (-7.1692, -0.9745) (-7.1589, -0.9792) (-7.1485, -0.9838) (-7.1382, -0.9884) (-7.1279, -0.9929) (-7.1176, -0.9974) (-7.1074, -1.0018) (-7.0972, -1.0062) (-7.087, -1.0106) (-7.0768, -1.0149) (-7.0666, -1.0191) (-7.0565, -1.0233) (-7.0464, -1.0275) (-7.0363, -1.0316) (-7.0262, -1.0356) (-7.0162, -1.0397) (-7.0062, -1.0436) (-6.9962, -1.0476) (-6.9862, -1.0515) (-6.9763, -1.0553) (-6.9664, -1.0591) (-6.9565, -1.0628) (-6.9467, -1.0666) (-6.9368, -1.0702) (-6.927, -1.0738) (-6.9173, -1.0774) (-6.9075, -1.0809) (-6.8978, -1.0844) (-6.8881, -1.0879) (-6.8785, -1.0913) (-6.8689, -1.0946) (-6.8593, -1.0979) (-6.8497, -1.1012) (-6.8402, -1.1044) (-6.8307, -1.1076) (-6.8212, -1.1107) (-6.8118, -1.1138) (-6.8024, -1.1168) (-6.793, -1.1199) (-6.7837, -1.1228) (-6.7744, -1.1257) (-6.7651, -1.1286) (-6.7558, -1.1314) (-6.7466, -1.1342) (-6.7375, -1.137) (-6.7283, -1.1397) (-6.7192, -1.1424) (-6.7102, -1.145) (-6.7011, -1.1476) (-6.6921, -1.1501) (-6.6832, -1.1526) (-6.6743, -1.1551) (-6.6654, -1.1575) (-6.6565, -1.1599) (-6.6477, -1.1622) (-6.639, -1.1645) (-6.6302, -1.1668) (-6.6216, -1.169) (-6.6129, -1.1712) (-6.6043, -1.1733) (-6.5957, -1.1754) (-6.5872, -1.1774) (-6.5787, -1.1795) (-6.5703, -1.1814) (-6.5619, -1.1834) (-6.5535, -1.1853) (-6.5452, -1.1872) (-6.5369, -1.189) (-6.5287, -1.1908) (-6.5205, -1.1925) (-6.5124, -1.1942) (-6.5043, -1.1959) (-6.4962, -1.1975) (-6.4882, -1.1991) (-6.4802, -1.2007) (-6.4723, -1.2022) (-6.4645, -1.2037) (-6.4566, -1.2052) (-6.4489, -1.2066) (-6.4411, -1.208) (-6.4335, -1.2093) (-6.4258, -1.2106) (-6.4183, -1.2119) (-6.4107, -1.2131) (-6.4033, -1.2144) (-6.3958, -1.2155) (-6.3885, -1.2167) (-6.3811, -1.2178) (-6.3739, -1.2188) (-6.3666, -1.2199) (-6.3595, -1.2209) (-6.3524, -1.2219) (-6.3453, -1.2228) (-6.3383, -1.2237) (-6.3314, -1.2246) (-6.3245, -1.2254) (-6.3176, -1.2262) (-6.3109, -1.227) (-6.3041, -1.2278) (-6.2975, -1.2285) (-6.2909, -1.2292) (-6.2843, -1.2299) (-6.2778, -1.2305) (-6.2714, -1.2311) (-6.265, -1.2317) (-6.2587, -1.2322) (-6.2525, -1.2327) (-6.2463, -1.2332) (-6.2402, -1.2337) (-6.2341, -1.2341) (-6.2281, -1.2346) (-6.2222, -1.2349) (-6.2163, -1.2353) (-6.2105, -1.2356) (-6.2048, -1.236) (-6.1991, -1.2362) (-6.1935, -1.2365) (-6.188, -1.2367) (-6.1825, -1.237) (-6.1771, -1.2372) (-6.1718, -1.2373) (-6.1665, -1.2375) (-6.1613, -1.2376) (-6.1562, -1.2377) (-6.1511, -1.2378) (-6.1462, -1.2379) (-6.1413, -1.2379) (-6.1364, -1.2379) (-6.1317, -1.2379) (-6.127, -1.2379) (-6.1224, -1.2379) (-6.1179, -1.2379) (-6.1134, -1.2378) (-6.109, -1.2377) (-6.1047, -1.2376) (-6.1005, -1.2375) (-6.0964, -1.2374) (-6.0923, -1.2373) (-6.0884, -1.2371) (-6.0845, -1.237) (-6.0807, -1.2368) (-6.077, -1.2366) (-6.0733, -1.2364) (-6.0698, -1.2362) (-6.0663, -1.236) (-6.0629, -1.2358) (-6.0596, -1.2356) (-6.0564, -1.2353) (-6.0533, -1.2351) (-6.0503, -1.2349) (-6.0474, -1.2346) (-6.0446, -1.2344) (-6.0418, -1.2341) (-6.0392, -1.2339) (-6.0366, -1.2336) (-6.0342, -1.2333) (-6.0318, -1.2331) (-6.0296, -1.2328) (-6.0274, -1.2326) (-6.0254, -1.2323) (-6.0234, -1.2321) (-6.0216, -1.2318) (-6.0198, -1.2316) (-6.0182, -1.2314) (-6.0166, -1.2311) (-6.0152, -1.2309) (-6.0139, -1.2307) (-6.0127, -1.2305) (-6.0116, -1.2304) (-6.0106, -1.2302) (-6.0098, -1.23) (-6.009, -1.2299) (-6.0085, -1.2298) (-6.0082, -1.2298) (-6.008, -1.2297) (-6.0079, -1.2297) knots -1 -1 -1 -1 -1 -1 -0.99583333 -0.99166667 -0.9875 -0.98333333 -0.97916667 -0.975 -0.97083333 -0.96666667 -0.9625 -0.95833333 -0.95416667 -0.95 -0.94583333 -0.94166667 -0.9375 -0.93333333 -0.92916667 -0.925 -0.92083333 -0.91666667 -0.9125 -0.90833333 -0.90416667 -0.9 -0.89583333 -0.89166667 -0.8875 -0.88333333 -0.87916667 -0.875 -0.87083333 -0.86666667 -0.8625 -0.85833333 -0.85416667 -0.85 -0.84583333 -0.84166667 -0.8375 -0.83333333 -0.82916667 -0.825 -0.82083333 -0.81666667 -0.8125 -0.80833333 -0.80416667 -0.8 -0.79583333 -0.79166667 -0.7875 -0.78333333 -0.77916667 -0.775 -0.77083333 -0.76666667 -0.7625 -0.75833333 -0.75416667 -0.75 -0.74583333 -0.74166667 -0.7375 -0.73333333 -0.72916667 -0.725 -0.72083333 -0.71666667 -0.7125 -0.70833333 -0.70416667 -0.7 -0.69583333 -0.69166667 -0.6875 -0.68333333 -0.67916667 -0.675 -0.67083333 -0.66666667 -0.6625 -0.65833333 -0.65416667 -0.65 -0.64583333 -0.64166667 -0.6375 -0.63333333 -0.62916667 -0.625 -0.62083333 -0.61666667 -0.6125 -0.60833333 -0.60416667 -0.6 -0.59583333 -0.59166667 -0.5875 -0.58333333 -0.57916667 -0.575 -0.57083333 -0.56666667 -0.5625 -0.55833333 -0.55416667 -0.55 -0.54583333 -0.54166667 -0.5375 -0.53333333 -0.52916667 -0.525 -0.52083333 -0.51666667 -0.5125 -0.50833333 -0.50416667 -0.5 -0.49583333 -0.49166667 -0.4875 -0.48333333 -0.47916667 -0.475 -0.47083333 -0.46666667 -0.4625 -0.45833333 -0.45416667 -0.45 -0.44583333 -0.44166667 -0.4375 -0.43333333 -0.42916667 -0.425 -0.42083333 -0.41666667 -0.4125 -0.40833333 -0.40416667 -0.4 -0.39583333 -0.39166667 -0.3875 -0.38333333 -0.37916667 -0.375 -0.37083333 -0.36666667 -0.3625 -0.35833333 -0.35416667 -0.35 -0.34583333 -0.34166667 -0.3375 -0.33333333 -0.32916667 -0.325 -0.32083333 -0.31666667 -0.3125 -0.30833333 -0.30416667 -0.3 -0.29583333 -0.29166667 -0.2875 -0.28333333 -0.27916667 -0.275 -0.27083333 -0.26666667 -0.2625 -0.25833333 -0.25416667 -0.25 -0.24583333 -0.24166667 -0.2375 -0.23333333 -0.22916667 -0.225 -0.22083333 -0.21666667 -0.2125 -0.20833333 -0.20416667 -0.2 -0.19583333 -0.19166667 -0.1875 -0.18333333 -0.17916667 -0.175 -0.17083333 -0.16666667 -0.1625 -0.15833333 -0.15416667 -0.15 -0.14583333 -0.14166667 -0.1375 -0.13333333 -0.12916667 -0.125 -0.12083333 -0.11666667 -0.1125 -0.10833333 -0.10416667 -0.1 -0.09583333 -0.09166667 -0.0875 -0.08333333 -0.07916667 -0.075 -0.07083333 -0.06666667 -0.0625 -0.05833333 -0.05416667 -0.05 -0.04583333 -0.04166667 -0.0375 -0.03333333 -0.02916667 -0.025 -0.02083333 -0.01666667 -0.0125 -0.00833333 -0.00416667 0 0 0 0 0 0
  line L2 (-6.0079, -1.2297) -> (-6.0071, -1.2295)
  line L3 (-6.0071, -1.2295) -> (-4.2657, -0.8731)
  arc A2 (-4.2657, -0.8731) -> (-3.6337, -2.3989) centre (0, 0) ccw
  line L4 (-3.6337, -2.3989) -> (-5.1171, -3.3782)
  line L5 (-5.1171, -3.3782) -> (-5.1178, -3.3787)
  spline S2 degree 5 poles (-5.1178, -3.3787) (-5.1178, -3.3787) (-5.118, -3.3789) (-5.1183, -3.379) (-5.1187, -3.3793) (-5.1193, -3.3798) (-5.12, -3.3803) (-5.1208, -3.3809) (-5.1217, -3.3815) (-5.1227, -3.3822) (-5.1238, -3.383) (-5.125, -3.3839) (-5.1262, -3.3848) (-5.1275, -3.3858) (-5.1289, -3.3869) (-5.1304, -3.388) (-5.1319, -3.3892) (-5.1336, -3.3905) (-5.1353, -3.3918) (-5.1371, -3.3932) (-5.1389, -3.3947) (-5.1408, -3.3963) (-5.1428, -3.3979) (-5.1449, -3.3996) (-5.147, -3.4013) (-5.1492, -3.4031) (-5.1514, -3.405) (-5.1537, -3.407) (-5.1561, -3.409) (-5.1585, -3.4111) (-5.161, -3.4133) (-5.1635, -3.4155) (-5.1661, -3.4178) (-5.1688, -3.4202) (-5.1715, -3.4226) (-5.1742, -3.4251) (-5.1771, -3.4277) (-5.1799, -3.4303) (-5.1828, -3.4331) (-5.1858, -3.4358) (-5.1888, -3.4387) (-5.1918, -3.4416) (-5.1949, -3.4445) (-5.1981, -3.4476) (-5.2013, -3.4507) (-5.2045, -3.4538) (-5.2078, -3.4571) (-5.2111, -3.4604) (-5.2145, -3.4638) (-5.2179, -3.4672) (-5.2213, -3.4707) (-5.2248, -3.4743) (-5.2283, -3.4779) (-5.2318, -3.4816) (-5.2354, -3.4853) (-5.239, -3.4892) (-5.2427, -3.4931) (-5.2463, -3.497) (-5.2501, -3.501) (-5.2538, -3.5051) (-5.2576, -3.5093) (-5.2614, -3.5135) (-5.2652, -3.5178) (-5.2691, -3.5221) (-5.273, -3.5265) (-5.2769, -3.531) (-5.2809, -3.5355) (-5.2848, -3.5401) (-5.2888, -3.5448) (-5.2929, -3.5495) (-5.2969, -3.5543) (-5.301, -3.5591) (-5.3051, -3.564) (-5.3092, -3.569) (-5.3133, -3.574) (-5.3175, -3.5791) (-5.3217, -3.5843) (-5.3259, -3.5895) (-5.3301, -3.5948) (-5.3343, -3.6002) (-5.3386, -3.6056) (-5.3429, -3.611) (-5.3472, -3.6166) (-5.3515, -3.6222) (-5.3558, -3.6278) (-5.3601, -3.6335) (-5.3645, -3.6393) (-5.3689, -3.6452) (-5.3732, -3.6511) (-5.3776, -3.657) (-5.382, -3.663) (-5.3865, -3.6691) (-5.3909, -3.6753) (-5.3953, -3.6815) (-5.3998, -3.6877) (-5.4043, -3.694) (-5.4087, -3.7004) (-5.4132, -3.7069) (-5.4177, -3.7134) (-5.4222, -3.7199) (-5.4267, -3.7265) (-5.4312, -3.7332) (-5.4358, -3.7399) (-5.4403, -3.7467) (-5.4448, -3.7536) (-5.4494, -3.7605) (-5.4539, -3.7675) (-5.4585, -3.7745) (-5.463, -3.7816) (-5.4676, -3.7887) (-5.4722, -3.7959) (-5.4767, -3.8032) (-5.4813, -3.8105) (-5.4859, -3.8178) (-5.4904, -3.8253) (-5.495, -3.8328) (-5.4996, -3.8403) (-5.5042, -3.8479) (-5.5087, -3.8556) (-5.5133, -3.8633) (-5.5179, -3.871) (-5.5225, -3.8789) (-5.527, -3.8867) (-5.5316, -3.8947) (-5.5362, -3.9027) (-5.5408, -3.9107) (-5.5453, -3.9188) (-5.5499, -3.927) (-5.5544, -3.9352) (-5.559, -3.9434) (-5.5635, -3.9518) (-5.5681, -3.9601) (-5.5726, -3.9686) (-5.5772, -3.977) (-5.5817, -3.9856) (-5.5862, -3.9942) (-5.5907, -4.0028) (-5.5952, -4.0115) (-5.5997, -4.0203) (-5.6042, -4.0291) (-5.6087, -4.0379) (-5.6132, -4.0468) (-5.6177, -4.0558) (-5.6221, -4.0648) (-5.6266, -4.0739) (-5.631, -4.083) (-5.6355, -4.0922) (-5.6399, -4.1014) (-5.6443, -4.1107) (-5.6487, -4.12) (-5.6531, -4.1294) (-5.6575, -4.1389) (-5.6618, -4.1483) (-5.6662, -4.1579) (-5.6705, -4.1675) (-5.6749, -4.1771) (-5.6792, -4.1868) (-5.6835, -4.1965) (-5.6878, -4.2063) (-5.6921, -4.2162) (-5.6964, -4.226) (-5.7006, -4.236) (-5.7048, -4.246) (-5.7091, -4.256) (-5.7133, -4.2661) (-5.7175, -4.2762) (-5.7217, -4.2864) (-5.7258, -4.2967) (-5.73, -4.307) (-5.7341, -4.3173) (-5.7382, -4.3277) (-5.7423, -4.3381) (-5.7464, -4.3486) (-5.7504, -4.3591) (-5.7545, -4.3697) (-5.7585, -4.3803) (-5.7625, -4.391) (-5.7665, -4.4017) (-5.7705, -4.4125) (-5.7744, -4.4233) (-5.7784, -4.4341) (-5.7823, -4.445) (-5.7862, -4.456) (-5.7901, -4.467) (-5.7939, -4.478) (-5.7978, -4.4891) (-5.8016, -4.5003) (-5.8054, -4.5114) (-5.8091, -4.5227) (-5.8129, -4.5339) (-5.8166, -4.5453) (-5.8203, -4.5566) (-5.824, -4.568) (-5.8277, -4.5795) (-5.8313, -4.591) (-5.835, -4.6025) (-5.8386, -4.6141) (-5.8421, -4.6258) (-5.8457, -4.6374) (-5.8492, -4.6492) (-5.8527, -4.6609) (-5.8562, -4.6727) (-5.8596, -4.6846) (-5.8631, -4.6965) (-5.8665, -4.7084) (-5.8699, -4.7204) (-5.8732, -4.7324) (-5.8766, -4.7445) (-5.8799, -4.7566) (-5.8832, -4.7688) (-5.8864, -4.7809) (-5.8896, -4.7932) (-5.8928, -4.8055) (-5.896, -4.8178) (-5.8992, -4.8301) (-5.9023, -4.8425) (-5.9054, -4.855) (-5.9085, -4.8675) (-5.9115, -4.88) (-5.9145, -4.8926) (-5.9175, -4.9052) (-5.9205, -4.9178) (-5.9234, -4.9305) (-5.9263, -4.9432) (-5.9292, -4.956) (-5.932, -4.9688) (-5.9349, -4.9817) (-5.9377, -4.9945) (-5.9404, -5.0075) (-5.9432, -5.0204) (-5.9459, -5.0334) (-5.9485, -5.0465) (-5.9512, -5.0596) (-5.9538, -5.0727) (-5.9564, -5.0858) (-5.9589, -5.099) (-5.9614, -5.1123) (-5.9639, -5.1255) (-5.9664, -5.1389) (-5.9688, -5.1522) (-5.9712, -5.1656) (-5.9731, -5.1763) (-5.9745, -5.1844) (-5.9755, -5.1898) (-5.9759, -5.1925) knots 0 0 0 0 0 0 0.00416667 0.00833333 0.0125 0.01666667 0.02083333 0.025 0.02916667 0.03333333 0.0375 0.04166667 0.04583333 0.05 0.05416667 0.05833333 0.0625 0.06666667 0.07083333 0.075 0.07916667 0.08333333 0.0875 0.09166667 0.09583333 0.1 0.10416667 0.10833333 0.1125 0.11666667 0.12083333 0.125 0.12916667 0.13333333 0.1375 0.14166667 0.14583333 0.15 0.15416667 0.15833333 0.1625 0.16666667 0.17083333 0.175 0.17916667 0.18333333 0.1875 0.19166667 0.19583333 0.2 0.20416667 0.20833333 0.2125 0.21666667 0.22083333 0.225 0.22916667 0.23333333 0.2375 0.24166667 0.24583333 0.25 0.25416667 0.25833333 0.2625 0.26666667 0.27083333 0.275 0.27916667 0.28333333 0.2875 0.29166667 0.29583333 0.3 0.30416667 0.30833333 0.3125 0.31666667 0.32083333 0.325 0.32916667 0.33333333 0.3375 0.34166667 0.34583333 0.35 0.35416667 0.35833333 0.3625 0.36666667 0.37083333 0.375 0.37916667 0.38333333 0.3875 0.39166667 0.39583333 0.4 0.40416667 0.40833333 0.4125 0.41666667 0.42083333 0.425 0.42916667 0.43333333 0.4375 0.44166667 0.44583333 0.45 0.45416667 0.45833333 0.4625 0.46666667 0.47083333 0.475 0.47916667 0.48333333 0.4875 0.49166667 0.49583333 0.5 0.50416667 0.50833333 0.5125 0.51666667 0.52083333 0.525 0.52916667 0.53333333 0.5375 0.54166667 0.54583333 0.55 0.55416667 0.55833333 0.5625 0.56666667 0.57083333 0.575 0.57916667 0.58333333 0.5875 0.59166667 0.59583333 0.6 0.60416667 0.60833333 0.6125 0.61666667 0.62083333 0.625 0.62916667 0.63333333 0.6375 0.64166667 0.64583333 0.65 0.65416667 0.65833333 0.6625 0.66666667 0.67083333 0.675 0.67916667 0.68333333 0.6875 0.69166667 0.69583333 0.7 0.70416667 0.70833333 0.7125 0.71666667 0.72083333 0.725 0.72916667 0.73333333 0.7375 0.74166667 0.74583333 0.75 0.75416667 0.75833333 0.7625 0.76666667 0.77083333 0.775 0.77916667 0.78333333 0.7875 0.79166667 0.79583333 0.8 0.80416667 0.80833333 0.8125 0.81666667 0.82083333 0.825 0.82916667 0.83333333 0.8375 0.84166667 0.84583333 0.85 0.85416667 0.85833333 0.8625 0.86666667 0.87083333 0.875 0.87916667 0.88333333 0.8875 0.89166667 0.89583333 0.9 0.90416667 0.90833333 0.9125 0.91666667 0.92083333 0.925 0.92916667 0.93333333 0.9375 0.94166667 0.94583333 0.95 0.95416667 0.95833333 0.9625 0.96666667 0.97083333 0.975 0.97916667 0.98333333 0.9875 0.99166667 0.99583333 1 1 1 1 1 1
  arc A3 (-5.9759, -5.1925) -> (-5.1925, -5.9759) centre (0, 0) ccw